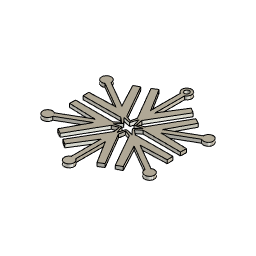
Snowflake 6 (Autodesk Fusion 360 design; units mm, degrees)
Autodesk Fusion 360 part; units mm, degrees
note: some values were not read from the file. Set by a fixed rule: which sketch regions a step uses.
sketch "Sketch1" plane through (0, 0, 0) normal (0, 0, 1) x (1, 0, 0)
  line L0 (-4.5, 24) -> (4.5, 24)
  line L1 (4.5, 112) -> (-4.5, 112)
  line L2 (-4.5, 112) -> (-4.5, 24)
  line L3 (0, 24) -> (0, 112) construction
  line L4 (4.5, 112) -> (4.5, 24)
  line L5 (0, 24) -> (0, 0) construction
  circle A0 centre (0, 120.9303) radius 10
  dimension "d517" = 9
  dimension "d518" = 88
  dimension "d519" = 24
  dimension "d520" = 20
  constraint horizontal L0
  constraint midpoint L0 L3.start
  constraint midpoint L1 L3.end
  constraint horizontal L1
  constraint vertical L4
  constraint vertical L2
  constraint coincident L5.end origin
  constraint vertical L5
  constraint coincident L1.start A0
  constraint coincident L1.end A0
  measures "d517" distance of L0.start L0.end
  measures "d518" distance of L0.end L1.start
  measures "d519" distance of L5.end L0
  measures "d520" diameter of A0
extrude "Extrude1" add sketch "Sketch1" along normal blind 7 makes body 1
sketch "Sketch2" plane through (0, 0, 0) normal (0, 0, 1) x (1, 0, 0)
  arc A0 (4.5, 112) -> (-4.5, 112) centre (0, 120.9303) ccw construction
  line L0 (4.5, 112) -> (4.5, 24) construction
  line L1 (4.5, 24) -> (-4.5, 24) construction
  line L2 (-4.5, 24) -> (-4.5, 112) construction
  line L3 (4.5, 51.0811) -> (33.1156, 96.8757)
  line L4 (33.1156, 96.8757) -> (43.3486, 90.4815)
  line L5 (43.3486, 90.4815) -> (4.5, 24)
  line L6 (4.5, 24) -> (4.5, 51.0811)
  dimension "d525" = 54
  dimension "d526" = 32
  dimension "d527" = 1.7
  dimension "d528" = 77
  constraint coincident L0 L3.start
  constraint coincident L0.end L1.start
  constraint perpendicular L3 L4
  measures "d525" distance of L3.start L3.end
  measures "d526" angle of L3 L6
  measures "d527" angle of L3 L5
  measures "d528" distance of L4.end L0.end
extrude "Extrude2" add sketch "Sketch2" along normal up to surface (7 mm away) separate body makes body 2
mirror "Mirror1" about plane through (0, 0, 0) normal (1, 0, 0) of bodies 2 makes body 3
combine "Combine1" operation add target body 2 tool bodies 1 3
sketch "Sketch3" plane through (0, 0, 0) normal (0, 0, 1) x (1, 0, 0)
  line L0 (43.3486, 90.4815) -> (4.5, 24)
  line L1 (4.5, 24) -> (-4.5, 24)
  line L2 (-4.5, 24) -> (-43.3486, 90.4815)
  line L3 (-43.3486, 90.4815) -> (-33.1156, 96.8757)
  line L4 (-33.1156, 96.8757) -> (-4.5, 51.0811)
  line L5 (-4.5, 51.0811) -> (-4.5, 112)
  arc A0 (4.5, 112) -> (-4.5, 112) centre (0, 120.9303) ccw
  line L6 (4.5, 112) -> (4.5, 51.0811)
  line L7 (4.5, 51.0811) -> (33.1156, 96.8757)
  line L8 (33.1156, 96.8757) -> (43.3486, 90.4815)
  line L9 (4.5, 24) -> (6.6025, 11.4359)
  line L10 (6.6025, 11.4359) -> (4.5525, 7.8852)
  line L11 (4.5525, 7.8852) -> (0, 22.1776)
  line L12 (0, 22.1776) -> (-4.5525, 7.8852)
  line L13 (-4.5525, 7.8852) -> (-6.6025, 11.4359)
  line L14 (-6.6025, 11.4359) -> (-4.5, 24)
  line L15 (0, 1.75) -> (0, 22.5)
  line L16 (1.75, 0) -> (22.5, 0)
  dimension "d533" = 60
  dimension "d538" = 15
  dimension "d539" = 4.1
  dimension "d540" = 19
  constraint coincident L0.end L1.start
  constraint coincident L1.end L2.start
  constraint vertical origin L11.end
  constraint symmetric L11 L12 L15
  constraint symmetric L9 L14 L15
  constraint symmetric L10 L13 L15
  constraint coincident origin L10
  constraint coincident origin L13
  measures "d533" angle of L10 L16
  measures "d538" distance of L10.end L11.end
  measures "d539" distance of L9.end L10.end
  measures "d540" angle of L9 L14
extrude "Extrude3" add sketch "Sketch3" along normal up to surface (7 mm away) separate body contours L1 L9 L10 L11 L12 L13 L14 makes body 4
pattern_circular "C-Pattern1" count 6 over 360 about axis through (0, 0, 1.75) along (0, 0, 1) of bodies 4 makes body 5 at (-14.7812, 12.8073, 0) makes body 6 at (-18.482, -6.3972, 0) makes body 7 at (-3.7008, -19.2045, 0) makes body 8 at (14.7812, -12.8073, 0) makes body 9 at (18.482, 6.3972, 0)
pattern_circular "C-Pattern2" count 6 over 360 about axis through (0, 0, 1.75) along (0, 0, 1) of bodies 2 makes body 10 at (-56.5186, 12.482, 7) makes body 11 at (-39.069, -42.7055, 7) makes body 12 at (17.4495, -55.1875, 0) makes body 13 at (56.5186, -12.482, 0) makes body 14 at (56.5186, 12.482, 7)
combine "Combine2" operation add target body 2 tool bodies 14 13 12 11 10 5 4 9 8 7 6
sketch "Sketch4" plane through (0, 0, 7) normal (0, 0, 1) x (-1, 0, 0)
  arc A0 (-4.5, -112) -> (4.5, -112) centre (0, -120.9303) ccw
  circle A1 centre (0, -120.9303) radius 5
  dimension "d543" = 10
  constraint concentric A0 A1
  measures "d543" diameter of A1
extrude "Extrude4" cut sketch "Sketch4" against normal up to surface (7 mm away) bodies 2
equation "d526 = 32.00 °"
equation "d527 = 1.7 °"
equation "d533 = ( 360 / 6 ) * 1 °"
equation "d540 = 19 °"
